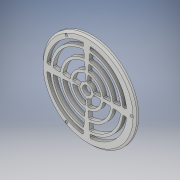
# Autodesk Inventor part: gimbalThrusterBackCover
Saved by Autodesk Inventor 2018 (Build 220112000, 112)
## iProperties
Created: 2020-01-26
Part Number: gimbalThrusterBackCover
Material: Generic
Document SubType Name: Modeling
Designer: anirudh
Density: 1 g/cm^3
Appearance: Default
Author: anirudh
Autodesk Inventor part; units mm, degrees
ref_plane "YZ Plane" through (0, 0, 0) normal (1, 0, 0) x (0, 1, 0)
ref_plane "XZ Plane" through (0, 0, 0) normal (0, 1, 0) x (-1, 0, 0)
ref_plane "XY Plane" through (0, 0, 0) normal (0, 0, 1) x (1, 0, 0)
sketch "Sketch2" plane through (0, 0, 0) normal (0, 0, 1) x (1, 0, 0)
  circle A0 centre (0, 0) radius 62.4586
  circle A1 centre (-1.8034, 0) radius 5.715
  dimension "d97" = 11.43
  constraints: 2 centre point, 2 coincident
  measures "d97" diameter of A1
ref_plane "Work Plane1" through (0, 0, 5.08) normal (0, 0, 1) x (1, 0, 0)
sketch "Sketch3" plane through (0, 0, 5.08) normal (0, 0, 1) x (1, 0, 0)
  circle A0 centre (0, 0) radius 62.4586 projected
  line L0 (0, 0) -> (57.8866, 0) construction
  circle A1 centre (-28.9433, 50.1313) radius 1.75
  circle A2 centre (-28.9433, -50.1313) radius 1.75
  circle A3 centre (57.8866, 0) radius 1.75
  dimension "d33" = 3.5
  dimension "d34" = 3.5
  dimension "d35" = 3.5
  constraints: 3 centre point, 2 end point, 1 coincident, 1 horizontal
  measures "d33" diameter of A1
  measures "d34" diameter of A2
  measures "d35" diameter of A3
extrude "Extrusion6" add sketch "Sketch2" along normal blind 5.08
extrude "Extrusion7" cut sketch "Sketch3" against normal blind 5.08 contours A1 | A2 | A3
sketch "Sketch6" plane through (0, 0, 0) normal (0, 0, -1) x (-1, 0, 0)
  arc A0 (1.0286, 8.8562) -> (-7.0528, 0.7748) centre (1.8034, 0) ccw
  arc A1 (0.157, 18.8181) -> (-17.0147, 1.6464) centre (1.8034, 0) ccw
  arc A2 (-0.1197, 21.981) -> (-20.1776, 1.9231) centre (1.8034, 0) ccw
  arc A3 (-0.9912, 31.943) -> (-30.1396, 2.7946) centre (1.8034, 0) ccw
  arc A4 (-1.268, 35.1059) -> (-33.3025, 3.0714) centre (1.8034, 0) ccw
  arc A5 (-2.1395, 45.0678) -> (-43.2644, 3.9429) centre (1.8034, 0) ccw
  arc A6 (-2.4162, 48.2308) -> (-46.4274, 4.2196) centre (1.8034, 0) ccw
  circle A7 centre (28.9433, 50.1313) radius 1.75 projected
  arc A8 (-2.8462, 53.1457) -> (-51.3423, 4.6496) centre (1.8034, 0) ccw
  line L0 (1.8034, 0) -> (67.9578, 0) construction
  circle A9 centre (1.8034, 0) radius 5.715 projected
  line L1 (1.8034, 0) -> (76.2837, 0) construction
  line L2 (-46.4274, 4.2196) -> (-51.3423, 4.6496)
  line L3 (-33.3025, 3.0714) -> (-43.2644, 3.9429)
  line L4 (-20.1776, 1.9231) -> (-30.1396, 2.7946)
  line L5 (-2.4162, 48.2308) -> (-2.8462, 53.1457)
  line L6 (-1.268, 35.1059) -> (-2.1395, 45.0678)
  line L7 (-0.1197, 21.981) -> (-0.9912, 31.943)
  line L8 (1.0286, 8.8562) -> (0.157, 18.8181)
  line L9 (-7.0528, 0.7748) -> (-17.0147, 1.6464)
  arc A10 (-51.3423, -4.6496) -> (-2.8462, -53.1457) centre (1.8034, 0) ccw
  arc A11 (-46.4274, -4.2196) -> (-2.4162, -48.2308) centre (1.8034, 0) ccw
  line L10 (-2.4162, -48.2308) -> (-2.8462, -53.1457)
  arc A12 (-43.2644, -3.9429) -> (-2.1395, -45.0678) centre (1.8034, 0) ccw
  line L11 (-1.268, -35.1059) -> (-2.1395, -45.0678)
  arc A13 (-33.3025, -3.0714) -> (-1.268, -35.1059) centre (1.8034, 0) ccw
  arc A14 (-30.1396, -2.7946) -> (-0.9912, -31.943) centre (1.8034, 0) ccw
  arc A15 (-20.1776, -1.9231) -> (-0.1197, -21.981) centre (1.8034, 0) ccw
  line L12 (-0.1197, -21.981) -> (-0.9912, -31.943)
  arc A16 (-17.0147, -1.6464) -> (0.157, -18.8181) centre (1.8034, 0) ccw
  arc A17 (-7.0528, -0.7748) -> (1.0286, -8.8562) centre (1.8034, 0) ccw
  line L13 (1.0286, -8.8562) -> (0.157, -18.8181)
  line L14 (-7.0528, -0.7748) -> (-17.0147, -1.6464)
  line L15 (-20.1776, -1.9231) -> (-30.1396, -2.7946)
  line L16 (-33.3025, -3.0714) -> (-43.2644, -3.9429)
  line L17 (-46.4274, -4.2196) -> (-51.3423, -4.6496)
  arc A18 (6.453, -53.1457) -> (54.9491, -4.6496) centre (1.8034, 0) ccw
  arc A19 (6.023, -48.2308) -> (50.0342, -4.2196) centre (1.8034, 0) ccw
  line L18 (50.0342, -4.2196) -> (54.9491, -4.6496)
  arc A20 (5.7463, -45.0678) -> (46.8712, -3.9429) centre (1.8034, 0) ccw
  line L19 (36.9093, -3.0714) -> (46.8712, -3.9429)
  arc A21 (4.8748, -35.1059) -> (36.9093, -3.0714) centre (1.8034, 0) ccw
  arc A22 (4.598, -31.943) -> (33.7464, -2.7946) centre (1.8034, 0) ccw
  arc A23 (3.7265, -21.981) -> (23.7844, -1.9231) centre (1.8034, 0) ccw
  line L20 (23.7844, -1.9231) -> (33.7464, -2.7946)
  arc A24 (3.4498, -18.8181) -> (20.6215, -1.6464) centre (1.8034, 0) ccw
  arc A25 (2.5782, -8.8562) -> (10.6596, -0.7748) centre (1.8034, 0) ccw
  line L21 (10.6596, -0.7748) -> (20.6215, -1.6464)
  line L22 (2.5782, -8.8562) -> (3.4498, -18.8181)
  line L23 (3.7265, -21.981) -> (4.598, -31.943)
  line L24 (4.8748, -35.1059) -> (5.7463, -45.0678)
  line L25 (6.023, -48.2308) -> (6.453, -53.1457)
  arc A26 (54.9491, 4.6496) -> (6.453, 53.1457) centre (1.8034, 0) ccw
  arc A27 (50.0342, 4.2196) -> (6.023, 48.2308) centre (1.8034, 0) ccw
  line L26 (6.023, 48.2308) -> (6.453, 53.1457)
  arc A28 (46.8712, 3.9429) -> (5.7463, 45.0678) centre (1.8034, 0) ccw
  line L27 (4.8748, 35.1059) -> (5.7463, 45.0678)
  arc A29 (36.9093, 3.0714) -> (4.8748, 35.1059) centre (1.8034, 0) ccw
  arc A30 (33.7464, 2.7946) -> (4.598, 31.943) centre (1.8034, 0) ccw
  arc A31 (23.7844, 1.9231) -> (3.7265, 21.981) centre (1.8034, 0) ccw
  line L28 (3.7265, 21.981) -> (4.598, 31.943)
  arc A32 (20.6215, 1.6464) -> (3.4498, 18.8181) centre (1.8034, 0) ccw
  arc A33 (10.6596, 0.7748) -> (2.5782, 8.8562) centre (1.8034, 0) ccw
  line L29 (2.5782, 8.8562) -> (3.4498, 18.8181)
  line L30 (10.6596, 0.7748) -> (20.6215, 1.6464)
  line L31 (23.7844, 1.9231) -> (33.7464, 2.7946)
  line L32 (36.9093, 3.0714) -> (46.8712, 3.9429)
  line L33 (50.0342, 4.2196) -> (54.9491, 4.6496)
  point P0 (0, 0)
  dimension "d114" = 360
  constraints: 68 end point, 64 point on circle, 32 centre point, 29 coincident, 2 horizontal, 161 other
extrude "Extrusion8" cut sketch "Sketch6" against normal blind 5.08 contours A0 L9 A1 L8 | A2 L4 A3 L7 | A4 L3 A5 L6 | A6 L2 A8 L5 | L17 A11 L10 A10 | L16 A13 L11 A12 | L15 A15 L12 A14 | L14 A17 L13 A16 | L25 A19 L18 A18 | L24 A21 L19 A20 | L23 A23 L20 A22 | L22 A25 L21 A24 | L33 A27 L26 A26 | L32 A29 L27 A28 | L31 A31 L28 A30 | L30 A33 L29 A32
fillet "Fillet5" radius 1.27 64 edges at (-54.9491, 4.6496, 2.54) (-50.0342, 4.2196, 2.54) (-6.453, 53.1457, 2.54) (-6.023, 48.2308, 2.54) (-5.7463, 45.0678, 2.54) (-4.8748, 35.1059, 2.54) (-46.8712, 3.9429, 2.54) (-36.9093, 3.0714, 2.54) (-33.7464, 2.7946, 2.54) (-23.7844, 1.9231, 2.54) (-3.7265, 21.981, 2.54) (-4.598, 31.943, 2.54) (-3.4498, 18.8181, 2.54) (-2.5782, 8.8562, 2.54) (-10.6596, 0.7748, 2.54) (-20.6215, 1.6464, 2.54) (-1.0286, 8.8562, 2.54) (-0.157, 18.8181, 2.54) (0.1197, 21.981, 2.54) (0.9912, 31.943, 2.54) (1.268, 35.1059, 2.54) (2.1395, 45.0678, 2.54) (2.4162, 48.2308, 2.54) (2.8462, 53.1457, 2.54) (51.3423, 4.6496, 2.54) (46.4274, 4.2196, 2.54) (43.2644, 3.9429, 2.54) (33.3025, 3.0714, 2.54) (30.1396, 2.7946, 2.54) (20.1776, 1.9231, 2.54) (17.0147, 1.6464, 2.54) (7.0528, 0.7748, 2.54) (7.0528, -0.7748, 2.54) (17.0147, -1.6464, 2.54) (20.1776, -1.9231, 2.54) (30.1396, -2.7946, 2.54) (33.3025, -3.0714, 2.54) (43.2644, -3.9429, 2.54) (46.4274, -4.2196, 2.54) (51.3423, -4.6496, 2.54) (2.8462, -53.1457, 2.54) (2.4162, -48.2308, 2.54) (2.1395, -45.0678, 2.54) (1.268, -35.1059, 2.54) (0.9912, -31.943, 2.54) (0.1197, -21.981, 2.54) (-0.157, -18.8181, 2.54) (-1.0286, -8.8562, 2.54) (-2.5782, -8.8562, 2.54) (-3.4498, -18.8181, 2.54) (-3.7265, -21.981, 2.54) (-4.598, -31.943, 2.54) (-4.8748, -35.1059, 2.54) (-5.7463, -45.0678, 2.54) (-6.023, -48.2308, 2.54) (-6.453, -53.1457, 2.54) (-54.9491, -4.6496, 2.54) (-50.0342, -4.2196, 2.54) (-46.8712, -3.9429, 2.54) (-36.9093, -3.0714, 2.54) (-33.7464, -2.7946, 2.54) (-23.7844, -1.9231, 2.54) (-20.6215, -1.6464, 2.54) (-10.6596, -0.7748, 2.54)
chamfer "Chamfer2" distance 2.54 angle 45 1 edges at (-62.4586, 0, 5.08)
body "Solid2"
